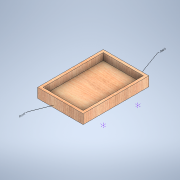
# Autodesk Inventor part: Part1proj
Saved by Autodesk Inventor 2020 (Build 240168000, 168)
## iProperties
Created: 2020-03-23
Part Number: Part1proj
Material: Wood (Birch)
Document SubType Name: Modeling
Designer: Manish
Density: 0.55 g/cm^3
Appearance: Birch - Natural Polished
Author: Manish
Autodesk Inventor part; units mm, degrees
ref_plane "YZ Plane" through (0, 0, 0) normal (1, 0, 0) x (0, 1, 0)
ref_plane "XZ Plane" through (0, 0, 0) normal (0, 1, 0) x (-1, 0, 0)
ref_plane "XY Plane" through (0, 0, 0) normal (0, 0, 1) x (1, 0, 0)
sketch "Sketch1" plane through (0, 0, 0) normal (0, 1, 0) x (-1, 0, 0)
  line L0 (7.9003, 23.0254) -> (-242.0997, 23.0254)
  line L1 (-242.0997, 23.0254) -> (-242.0997, -336.9746)
  line L2 (-242.0997, -336.9746) -> (7.9003, -336.9746)
  line L3 (7.9003, -336.9746) -> (7.9003, 23.0254)
  point P0 (0, 0)
  dimension "d0" = 250
  dimension "d1" = 360
  constraints: 8 end point, 2 parallel, 1 horizontal, 1 perpendicular
  measures "d0" distance of L2.end L1.end
  measures "d1" distance of L1.end L0.end
extrude "Extrusion1" add sketch "Sketch1" along normal blind 52
shell "Shell1" thickness 15 removed faces 1 at (158.7664, 52, -96.9746)
sketch3d "3D Sketch5"
body "Solid1"
